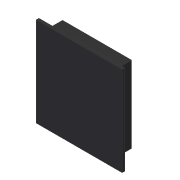
# Autodesk Inventor part: motor_mount_fitcheck1
Saved by Autodesk Inventor 2017 (Build 210142000, 142)
## iProperties
Created: 2018-10-28
Part Number: motor_mount_fitcheck1
Material: Generic
Document SubType Name: Modeling
Designer: mfans
Density: 1 g/cm^3
Appearance: Default
Author: mfans
Autodesk Inventor part; units mm, degrees
ref_plane "YZ Plane" through (0, 0, 0) normal (1, 0, 0) x (0, 1, 0)
ref_plane "XZ Plane" through (0, 0, 0) normal (0, 1, 0) x (-1, 0, 0)
ref_plane "XY Plane" through (0, 0, 0) normal (0, 0, 1) x (1, 0, 0)
sketch "Sketch1" plane through (0, 0, 0) normal (0, 1, 0) x (-1, 0, 0)
  line L0 (0, 0) -> (-14.5, 0)
  line L1 (-14.5, 0) -> (-14.5, -42.5)
  line L2 (-14.5, -42.5) -> (0, -42.5)
  line L3 (0, -42.5) -> (0, 0)
  line L4 (0, 0) -> (15.5, 0)
  line L5 (15.5, 0) -> (15.5, -17.25)
  line L6 (15.5, -17.25) -> (0, -17.25)
  line L7 (0, -17.25) -> (0, 0)
  line L8 (0, -17.25) -> (10, -17.25)
  line L9 (10, -17.25) -> (10, -18.25)
  line L10 (10, -18.25) -> (0, -18.25)
  line L11 (0, -18.25) -> (0, -17.25)
  line L12 (0, -17.25) -> (1, -17.25)
  line L13 (1, -17.25) -> (1, -27.25)
  line L14 (1, -27.25) -> (0, -27.25)
  line L15 (0, -27.25) -> (0, -17.25)
  line L16 (10, 0) -> (-14.5, 0)
  line L17 (-14.5, 0) -> (-14.5, 1)
  line L18 (-14.5, 1) -> (10, 1)
  line L19 (10, 1) -> (10, 0)
  line L20 (-14.5, 1) -> (-15.5, 1)
  line L21 (-15.5, 1) -> (-15.5, -27.25)
  line L22 (-15.5, -27.25) -> (-14.5, -27.25)
  line L23 (-14.5, -27.25) -> (-14.5, 1)
  line L24 (11.7177, -28.7701) -> (-19.9895, -28.7701)
  line L25 (-19.9895, -28.7701) -> (-19.9895, 4.2767)
  line L26 (-19.9895, 4.2767) -> (11.7177, 4.2767)
  line L27 (11.7177, 4.2767) -> (11.7177, -28.7701)
  dimension "d0" = 15.5
  dimension "d1" = 17.25
  dimension "d2" = 14.5
  dimension "d3" = 42.5
  dimension "d4" = 1
  dimension "d5" = 10
  dimension "d6" = 10
  dimension "d7" = 1
  dimension "d8" = 1
  dimension "d9" = 1
  dimension "d10" = 28.25
  constraints: 56 end point, 14 parallel, 7 horizontal, 7 perpendicular, 1 point on line
  measures "d0" distance between parallel lines of L3 L5
  measures "d1" distance of L4.end L5.end
  measures "d2" distance of L1.end L2.end
  measures "d3" distance of L0.end L1.end
  measures "d4" distance between parallel lines of L6 L10
  measures "d5" distance of L9.end L10.end
  measures "d6" distance of L12.end L13.end
  measures "d7" distance of L13.end L14.end
  measures "d8" distance of L16.end L17.end
  measures "d9" distance between parallel lines of L1 L21
  measures "d10" distance of L20.end L21.end
extrude "Extrusion1" add sketch "Sketch1" against normal blind 1 contours L3 L24 L1 L0 | L4 L27 L6 L3 | L0 L17 L18 L19 L4 | L1 L22 L21 L20 L17 | L6 L13 L10 L3 | L19 L18 L20 L21 L22 L1 L24 L25 L26 L27 L4 | L10 L13 L14 L3 | L6 L9 L10 L13 | L14 L13 L10 L9 L6 L27 L24 L3
extrude "Extrusion2" add sketch "Sketch1" along normal blind 7 contours L0 L17 L18 L19 L4 | L1 L22 L21 L20 L17 | L6 L13 L10 L3 | L10 L13 L14 L3 | L6 L9 L10 L13
sketch "Sketch2" plane through (-10, 0, -17.25) normal (-1, 0, 0) x (0, 0, 1)
  line L0 (0, 0) -> (-1, 0) projected
  line L1 (0, 0) -> (0, 7) projected
  line L2 (-1, 7) -> (0, 7) projected
  line L3 (-1, 0) -> (-1, 7) projected
  line L4 (18.25, 0) -> (17.25, 0) projected
  line L5 (18.25, 0) -> (18.25, 7) projected
  line L6 (17.25, 7) -> (18.25, 7) projected
  line L7 (17.25, 0) -> (17.25, 7) projected
  arc A0 (0, 4.027) -> (17.25, 4.027) centre (8.625, 11.25) ccw
  line L8 (21.5267, 0) -> (-11.5201, 0) projected
  line L9 (17.25, 4.027) -> (17.25, 0)
  line L10 (17.25, 0) -> (0, 0)
  line L11 (0, 0) -> (0, 4.027)
  line L12 (0, 0) -> (0, 7) projected
  line L13 (0, 4.027) -> (0, 0)
  line L14 (0, 0) -> (17.25, 0)
  line L15 (17.25, 0) -> (17.25, 4.027)
  arc A1 (0, 4.027) -> (17.25, 4.027) centre (8.625, 11.25) ccw
  line L16 (17.25, 4.027) -> (17.25, 0)
  line L17 (17.25, 0) -> (0, 0)
  line L18 (0, 0) -> (0, 4.027)
  line L19 (0, 4.027) -> (0, 0)
  line L20 (0, 0) -> (8.625, 0)
  line L21 (8.625, 0) -> (17.25, 0)
  line L22 (-11.5201, 0) -> (21.5267, 0) projected
  line L23 (17.25, 0) -> (17.25, 4.027)
  dimension "d15" = 8.625
  dimension "d16" = 22.5
  constraints: 26 end point, 4 point on circle, 2 centre point, 2 collinear, 2 parallel, 2 perpendicular, 2 point on line, 2 tangent, 2 vertical, 1 concentric, 1 midpoint
  measures "d15" distance from line of L1 A0.centre
  measures "d16" diameter of A0
sketch "Sketch3" plane through (-10, 0, -17.25) normal (-1, 0, 0) x (0, 0, 1)
  line L0 (0, 0) -> (-1, 0) projected
  line L1 (0, 0) -> (0, 7) projected
  line L2 (-1, 7) -> (0, 7) projected
  line L3 (-1, 0) -> (-1, 7) projected
  line L4 (18.25, 0) -> (17.25, 0) projected
  line L5 (18.25, 0) -> (18.25, 7) projected
  line L6 (17.25, 7) -> (18.25, 7) projected
  line L7 (17.25, 0) -> (17.25, 7) projected
  line L8 (21.5267, 0) -> (-11.5201, 0) projected
  arc A0 (0, 4.1686) -> (17.25, 4.1686) centre (8.625, 11.007) ccw
  line L9 (-11.5201, 0) -> (21.5267, 0) projected
  line L10 (0, 0) -> (0, 7) projected
  line L11 (0, 4.1686) -> (0, 0)
  line L12 (0, 0) -> (8.625, 0)
  line L13 (18.25, 0) -> (17.25, 0) projected
  line L14 (8.625, 0) -> (17.25, 0)
  line L15 (17.25, 0) -> (17.25, 4.1686)
  dimension "d17" = 8.625
  constraints: 8 end point, 3 point on circle, 3 point on line, 1 centre point, 1 horizontal, 1 tangent, 1 vertical
  measures "d17" distance from line of L1 A0.centre
extrude "Extrusion3" add sketch "Sketch3" against normal blind 10 contours A0 L7 L8 | L1 A0 L8
body "Solid1"
